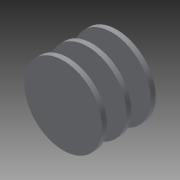
# Autodesk Inventor part: Spool
Saved by Autodesk Inventor 2015 SP1 (Build 190203100, 203)
## iProperties
Created: 2015-03-14
Part Number: Spool
Material: Generic
Document SubType Name: Modeling
Designer: fuji
Density: 1 g/cm^3
Appearance: Default
Author: fuji
Autodesk Inventor part; units mm, degrees
ref_plane "YZ Plane" through (0, 0, 0) normal (1, 0, 0) x (0, 1, 0)
ref_plane "XZ Plane" through (0, 0, 0) normal (0, 1, 0) x (-1, 0, 0)
ref_plane "XY Plane" through (0, 0, 0) normal (0, 0, 1) x (1, 0, 0)
sketch "Sketch1" plane through (0, 0, 0) normal (0, 0, 1) x (1, 0, 0)
  circle A0 centre (0, 0) radius 12.7
  dimension "d0" = 25.4
  constraints: 1 centre point, 1 coincident
  measures "d0" diameter of A0
extrude "Extrusion1" add sketch "Sketch1" along normal blind 1.5875
sketch "Sketch2" plane through (0, 0, 1.5875) normal (0, 0, 1) x (1, 0, 0)
  circle A0 centre (0, 0) radius 3.175
  dimension "d3" = 6.35
  constraints: 1 centre point, 1 coincident
  measures "d3" diameter of A0
extrude "Extrusion2" add sketch "Sketch2" along normal blind 6.35
sketch "Sketch3" plane through (0, 0, 7.9375) normal (0, 0, 1) x (1, 0, 0)
  circle A0 centre (0, 0) radius 12.7
  dimension "d6" = 25.4
  constraints: 1 centre point, 1 coincident
  measures "d6" diameter of A0
extrude "Extrusion3" add sketch "Sketch3" along normal blind 1.5875
sketch "Sketch4" plane through (0, 0, 9.525) normal (0, 0, 1) x (1, 0, 0)
  circle A0 centre (0, 0) radius 3.175
  dimension "d9" = 6.35
  constraints: 1 centre point, 1 coincident
  measures "d9" diameter of A0
extrude "Extrusion4" add sketch "Sketch4" along normal blind 6.35
sketch "Sketch5" plane through (0, 0, 15.875) normal (0, 0, 1) x (1, 0, 0)
  circle A0 centre (0, 0) radius 12.7
  dimension "d12" = 25.4
  constraints: 1 centre point, 1 coincident
  measures "d12" diameter of A0
extrude "Extrusion5" add sketch "Sketch5" along normal blind 1.5875
equation "\"d0\" = spoolD"
equation "\"d1\" = spoolT"
equation "\"d3\" = hubD"
equation "\"d4\" = hubH"
equation "\"d6\" = spoolD"
equation "\"d7\" = spoolT"
equation "\"d9\" = hubD"
equation "\"d10\" = hubH"
equation "\"d12\" = spoolD"
equation "\"d13\" = spoolT"
equation "\"spoolD\" = 25.4"
equation "\"hubD\" = 6.35"
equation "\"spoolT\" = 1.5875"
equation "\"hubH\" = 6.35"
equation "\"hornT\" = 1.5875"
equation "\"hornD\" = 25.4"
equation "\"hornS\" = 2.794"
equation "\"hornOD\" = 8.89"
equation "\"hornH\" = 2.54"
equation "\"hornID\" = 6.096"
equation "\"inset\" = 2.032"
equation "\"insetD\" = 5.842"
equation "\"servW\" = 20.1168"
equation "\"servL\" = 40.5892"
equation "\"servML\" = 49.784"
equation "\"servMW\" = 10.033"
equation "\"servMD\" = 3.175"
equation "\"housL\" = 53.975"
equation "\"housW\" = 28.575"
equation "\"housT\" = 2.54"
equation "\"housBT\" = 1.5875"
equation "\"housH\" = 39.116"
equation "\"guideW\" = 9.144"
equation "\"guideH\" = 23.114"
equation "\"guideD\" = 3.175"
body "Solid1"
